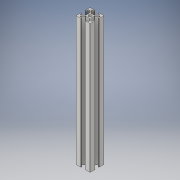
# Autodesk Inventor part: Profile_30mm_275mm
Saved by Autodesk Inventor 2018 (Build 220112000, 112)
## iProperties
Created: 2017-09-02
Part Number: Profile_30mm_275mm
Material: Generic
Document SubType Name: Modeling
Designer: snipe
Density: 1 g/cm^3
Appearance: Default
Author: snipe
Autodesk Inventor part; units mm, degrees
ref_plane "YZ Plane" through (0, 0, 0) normal (1, 0, 0) x (0, 1, 0)
ref_plane "XZ Plane" through (0, 0, 0) normal (0, 1, 0) x (-1, 0, 0)
ref_plane "XY Plane" through (0, 0, 0) normal (0, 0, 1) x (1, 0, 0)
sketch "Sketch1" plane through (0, 0, 0) normal (0, 1, 0) x (-1, 0, 0)
  line L0 (0, -21.0136) -> (0, 21.0817) projected
  line L1 (-21, 0) -> (21, 0) projected
  line L2 (21, 0) -> (-21, 0) projected
  line L3 (0, -21.0136) -> (0, 21.0817) projected
  line L4 (3.6865, 5.4825) -> (-4.0965, 5.4825)
  line L5 (-5.4825, 3.7546) -> (-5.4825, -4.0284)
  line L6 (-4.0967, -5.4144) -> (3.6863, -5.4144)
  line L7 (5.4825, -4.0284) -> (5.4825, 3.7546)
  line L8 (-5.4825, 5.4825) -> (5.4825, -5.4825) construction
  line L9 (15, 15.0681) -> (15, 4.2181)
  line L10 (15, 4.2181) -> (12.75, 4.2181)
  line L11 (15, 15.0681) -> (4.15, 15.0681)
  line L12 (4.15, 15.0681) -> (4.15, 12.8181)
  line L13 (-15, 14.795) -> (-4.15, 14.795)
  line L14 (-4.15, 14.795) -> (-4.15, 12.75)
  line L15 (-15, 12.75) -> (-15, 14.795)
  line L16 (-15, 14.795) -> (-12.75, 14.795)
  line L17 (-12.75, 3.945) -> (-15, 3.945)
  line L18 (-15, 3.945) -> (-15, 14.795)
  line L19 (-15, -14.9319) -> (-12.75, -14.9319)
  line L20 (-12.75, -4.0819) -> (-15, -4.0819)
  line L21 (-15, -4.0819) -> (-15, -14.9319)
  line L22 (-15, -14.9319) -> (-4.1502, -14.9319)
  line L23 (-4.1502, -14.9319) -> (-4.1502, -12.6819)
  line L24 (-15, -12.7481) -> (-15, -14.9319)
  line L25 (15, -14.9319) -> (12.75, -14.9319)
  line L26 (12.75, -4.0819) -> (15, -4.0819)
  line L27 (15, -4.0819) -> (15, -14.9319)
  line L28 (15, -14.9319) -> (4.1502, -14.9319)
  line L29 (4.1502, -14.9319) -> (4.1502, -12.6819)
  line L30 (15, -12.7481) -> (15, -14.9319)
  circle A0 centre (0, 0) radius 3.1425
  line L31 (8.9925, -14.9319) -> (4.1502, -14.9319)
  line L32 (-4.1502, -14.9319) -> (-8.9925, -14.9319)
  line L33 (15, -14.9319) -> (4.1502, -14.9319)
  line L34 (-4.1502, -14.9319) -> (-15, -14.9319)
  line L35 (15, -8.9925) -> (15, -4.0819)
  line L36 (15, 4.2181) -> (15, 9.0606)
  line L37 (15, 15.0681) -> (15, 4.2181)
  line L38 (15, -4.0819) -> (15, -14.9319)
  line L39 (-8.9925, 14.795) -> (-4.15, 14.795)
  line L40 (4.15, 15.0681) -> (8.9925, 15.0681)
  line L41 (-15, 14.795) -> (-4.15, 14.795)
  line L42 (4.15, 15.0681) -> (15, 15.0681)
  line L43 (-15, 8.9925) -> (-15, 3.945)
  line L44 (-15, -4.0819) -> (-15, -8.9925)
  line L45 (-15, -14.9319) -> (-15, -4.0819)
  line L46 (-15, 3.945) -> (-15, 14.795)
  line L47 (-4.1502, -12.6819) -> (-9.1977, -12.6819)
  line L48 (-12.75, -9.1294) -> (-12.75, -4.0819)
  line L49 (-12.75, -9.1294) -> (-10.5835, -9.1294)
  line L50 (-9.1977, -12.6819) -> (-9.1977, -10.5154)
  line L51 (-9.1975, 10.5835) -> (-9.1975, 12.75)
  line L52 (4.15, 12.8181) -> (8.7875, 12.8181)
  line L53 (12.75, 4.2181) -> (12.75, 8.8556)
  line L54 (12.75, 8.8556) -> (10.5835, 8.8556)
  line L55 (8.7875, 12.8181) -> (8.7875, 10.5835)
  line L56 (4.1502, -12.6819) -> (8.7873, -12.6819)
  line L57 (14.341, -12.7481) -> (15, -12.7481)
  line L58 (12.75, -14.9319) -> (12.75, -14.2729)
  line L59 (12.75, -9.1294) -> (12.75, -4.0819)
  line L60 (10.5835, -9.1294) -> (12.75, -9.1294)
  line L61 (8.7873, -10.5154) -> (8.7873, -12.6819)
  line L62 (5.4825, 5.4825) -> (-0.7955, -0.7955) construction
  line L63 (-2.2221, -2.2221) -> (-5.4825, -5.4825) construction
  line L64 (-12.75, 14.795) -> (-12.75, 14.136)
  line L65 (-12.75, 8.8556) -> (-12.75, 3.945)
  line L66 (-4.15, 12.75) -> (-9.1975, 12.75)
  line L67 (-14.341, 12.75) -> (-15, 12.75)
  line L68 (-10.5835, 8.8556) -> (-12.75, 8.8556)
  line L69 (-5.4825, 3.7546) -> (-10.5835, 8.8556)
  line L70 (-4.0965, 5.4825) -> (-9.1975, 10.5835)
  line L71 (8.7875, 10.5835) -> (3.6865, 5.4825)
  line L72 (10.5835, 8.8556) -> (5.4825, 3.7546)
  line L73 (10.5835, -9.1294) -> (5.4825, -4.0284)
  line L74 (8.7873, -10.5154) -> (3.6863, -5.4144)
  line L75 (-4.0967, -5.4144) -> (-9.1977, -10.5154)
  line L76 (-5.4825, -4.0284) -> (-10.5835, -9.1294)
  line L77 (15, 15) -> (-15, -15) construction
  line L78 (-15, 15) -> (15, -15) construction
  point P0 (-15, 0)
  dimension "d26" = 6.285
  dimension "d0" = 30
  dimension "d1" = 30
  dimension "d2" = 10.965
  dimension "d3" = 10.965
  dimension "d4" = 30
  dimension "d5" = 17.985
  dimension "d6" = 17.985
  dimension "d11" = 10.85
  dimension "d12" = 2.25
  dimension "d13" = 10.85
  dimension "d14" = 2.25
  dimension "d15" = 10.85
  dimension "d16" = 2.25
  dimension "d17" = 10.85
  dimension "d18" = 2.25
  dimension "d19" = 10.85
  dimension "d20" = 10.85
  dimension "d21" = 2.25
  dimension "d22" = 2.25
  dimension "d23" = 10.85
  dimension "d24" = 10.85
  dimension "d25" = 2.25
  dimension "d31" = 30
  dimension "d32" = 30
  constraints: 150 end point, 42 parallel, 28 perpendicular, 13 horizontal, 1 midpoint, 1 point on line, 3 other
  measures "d0" distance of L34.end L33.start
  measures "d1" distance of L33.start L9.start
  measures "d2" distance of L63.end L8.end
  measures "d3" distance of L8.start L63.end
  measures "d4" distance of L35.start L44.end
  measures "d5" distance of L44.end L43.start
  measures "d6" distance of L31.start L32.end
  measures "d11" distance of L9.end L9.start
  measures "d12" distance of L9.end L10.end
  measures "d13" distance of L9.start L11.end
  measures "d14" distance of L11.end L12.end
  measures "d15" distance of L14.end L15.start
  measures "d16" distance of L17.start L17.end
  measures "d17" distance of L16.end L17.start
  measures "d18" distance of L20.end L20.start
  measures "d19" distance of L20.start L19.end
  measures "d20" distance of L24.start L23.end
  measures "d21" distance of L23.end L22.end
  measures "d22" distance of L26.start L26.end
  measures "d23" distance of L25.end L26.start
  measures "d24" distance of L29.end L30.start
  measures "d25" distance of L28.end L29.end
  measures "d31" distance of L78.end L77.end
  measures "d32" distance of L77.end L78.start
extrude "Extrusion1" add sketch "Sketch1" along normal blind 275 contours L6 L75 L50 L47 L23 L22 L19 L21 L20 L48 L49 L76 L5 L1 A0 L0 | L0 A0 L1 L7 L73 L60 L59 L26 L27 L25 L28 L29 L56 L61 L74 L6 | L1 L5 L69 L68 L65 L17 L18 L15 L13 L14 L66 L51 L70 L4 L0 A0 | A0 L0 L4 L71 L55 L52 L12 L11 L9 L10 L53 L54 L72 L7 L1
fillet "Fillet1" radius 0.5 20 edges at (15, 137.5, 14.795) (4.15, 137.5, 14.795) (-4.15, 137.5, 15.0681) (-4.15, 137.5, 12.8181) (15, 137.5, 3.945) (12.75, 137.5, 3.945) (15, 137.5, -4.0819) (12.75, 137.5, -4.0819) (15, 137.5, -14.9319) (4.1502, 137.5, -12.6819) (-4.1502, 137.5, -14.9319) (-4.1502, 137.5, -12.6819) (4.1502, 137.5, -14.9319) (-15, 137.5, -14.9319) (-12.75, 137.5, -4.0819) (-15, 137.5, -4.0819) (-12.75, 137.5, 4.2181) (-15, 137.5, 4.2181) (-15, 137.5, 15.0681) (4.15, 137.5, 12.75)
fillet "Fillet2" radius 0.75 24 edges at (-10.5835, 137.5, 8.8556) (-5.4825, 137.5, 3.7546) (-12.75, 137.5, -9.1294) (-10.5835, 137.5, -9.1294) (-8.7873, 137.5, -12.6819) (5.4825, 137.5, -4.0284) (10.5835, 137.5, -9.1294) (-3.6865, 137.5, 5.4825) (-8.7875, 137.5, 10.5835) (5.4825, 137.5, 3.7546) (10.5835, 137.5, 8.8556) (12.75, 137.5, 8.8556) (12.75, 137.5, -9.1294) (4.0965, 137.5, 5.4825) (9.1975, 137.5, 10.5835) (9.1975, 137.5, 12.75) (-8.7875, 137.5, 12.8181) (-12.75, 137.5, 8.8556) (4.0967, 137.5, -5.4144) (9.1977, 137.5, -10.5154) (9.1977, 137.5, -12.6819) (-8.7873, 137.5, -10.5154) (-3.6863, 137.5, -5.4144) (-5.4825, 137.5, -4.0284)
body "Solid1"
